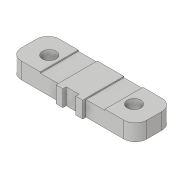
# Autodesk Inventor part: 8 peristaltic pump clamp 0.3mm
Saved by Autodesk Inventor 2020 (Build 240168000, 168)
## iProperties
Created: 2018-08-21
Part Number: 8 peristaltic pump clamp 0.3mm
Material: Generic
Document SubType Name: Modeling
Designer: mrbeh
Density: 1 g/cm^3
Appearance: Default
Author: mrbeh
Autodesk Inventor part; units mm, degrees
ref_plane "YZ Plane" through (0, 0, 0) normal (1, 0, 0) x (0, 1, 0)
ref_plane "XZ Plane" through (0, 0, 0) normal (0, 1, 0) x (-1, 0, 0)
sketch "Sketch1" plane through (0, 0, 0) normal (0, 1, 0) x (-1, 0, 0)
  line L0 (0, 0) -> (33, 0)
  line L1 (33, 0) -> (33, -10)
  line L2 (33, -10) -> (0, -10)
  line L3 (0, -10) -> (0, 0)
  dimension "d0" = 33
  dimension "d1" = 10
  constraints: 8 end point, 2 parallel, 1 horizontal, 1 perpendicular
  measures "d0" distance of L1.end L2.end
  measures "d1" distance of L0.end L1.end
extrude "Extrusion1" add sketch "Sketch1" along normal blind 4
sketch "Sketch2" plane through (0, 4, 0) normal (0, 1, 0) x (1, 0, 0)
  circle A0 centre (-5.343, 5) radius 1.8
  point P0 (0, 0)
  dimension "d9" = 3.6
  constraints: 1 centre point
  measures "d9" diameter of A0
extrude "Extrusion2" cut sketch "Sketch2" against normal blind 4
ref_plane "Work Plane1" through (-16.5, 0, 0) normal (1, 0, 0) x (0, 0, -1)
mirror "Mirror1" about plane through (-16.5, 0, 0) normal (1, 0, 0) of "Extrusion2"
fillet "Fillet1" radius 3 4 edges at (-33, 2, 0) (-33, 2, -10) (0, 2, 0) (0, 2, -10)
sketch "Sketch3" plane through (0, 4, 0) normal (0, 1, 0) x (1, 0, 0)
  line L0 (-30, 0) -> (-3, 0) projected
  line L1 (-30, 10) -> (-3, 10) projected
  line L2 (-20, 0) -> (-13, 0)
  line L3 (-13, 0) -> (-13, 10)
  line L4 (-13, 10) -> (-20, 10)
  line L5 (-20, 10) -> (-20, 0)
  point P0 (0, 0)
  dimension "d10" = 7
  dimension "d11" = 10
  constraints: 8 end point, 2 parallel, 1 horizontal, 1 perpendicular, 1 point on line
  measures "d10" distance of L4.end L3.end
  measures "d11" distance of L3.end L2.end
extrude "Extrusion3" add sketch "Sketch3" along normal blind 0.3
sketch "Sketch4" plane through (0, 4, 0) normal (0, 1, 0) x (1, 0, 0)
  line L0 (-3, 0) -> (-8, 0)
  line L1 (-8, 0) -> (-8, 10)
  line L2 (-8, 10) -> (-3, 10)
  line L3 (0, 7) -> (0, 3)
  arc A0 (-3, 0) -> (0, 3) centre (-3, 3) ccw
  arc A1 (0, 7) -> (-3, 10) centre (-3, 7) ccw
  circle A2 centre (-5.343, 5) radius 1.8 projected
  circle A3 centre (-5.343, 5) radius 1.8
  point P0 (0, 0)
  point P1 (0, 10)
  dimension "d14" = 8
  dimension "d15" = 10
  dimension "d16" = 3
  constraints: 8 end point, 4 point on circle, 4 point on line, 4 tangent, 3 centre point, 2 parallel, 1 coincident, 1 equal radius, 1 horizontal, 1 perpendicular
  measures "d14" distance of L1.end point (0, 10)
  measures "d15" distance of L0.end L1.end
  measures "d16" radius of A0
extrude "Extrusion4" add sketch "Sketch4" along normal blind 0.3
mirror "Mirror2" about plane through (-16.5, 0, 0) normal (1, 0, 0) of "Extrusion4"
sketch "Sketch6" plane through (0, 4.3, 0) normal (0, 1, 0) x (1, 0, 0)
  line L0 (-20, 0) -> (-13, 0) projected
  line L1 (-20, 0) -> (-18.2027, 0)
  line L2 (-18.2027, 0) -> (-18.2027, -0.8691)
  line L3 (-18.2027, -0.8691) -> (-20, -0.8691)
  line L4 (-20, -0.8691) -> (-20, 0)
  point P0 (0, 0)
  constraints: 8 end point, 2 parallel, 1 horizontal, 1 perpendicular
extrude "Extrusion6" add sketch "Sketch6" against normal up to surface (4.3 mm away)
sketch "Sketch7" plane through (0, 4.3, 0) normal (0, 1, 0) x (1, 0, 0)
  line L0 (-13, 0) -> (-13, 10) projected
  line L1 (-13, 0) -> (-14.8092, 0)
  line L2 (-14.8092, 0) -> (-14.8092, -0.8691)
  line L3 (-14.8092, -0.8691) -> (-13, -0.8691)
  line L4 (-13, -0.8691) -> (-13, 0)
  point P0 (0, 0)
  constraints: 8 end point, 2 parallel, 1 horizontal, 1 perpendicular
extrude "Extrusion7" add sketch "Sketch7" against normal up to surface (4.3 mm away)
body "Solid1"
